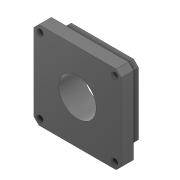
# Autodesk Inventor part: Front cover for servo motor 250 W
Saved by Autodesk Inventor 2020.3 (Build 243373010, 373A)
## iProperties
Created: 2021-04-26
Part Number: Front cover for servo motor 250 W
Material: PBT Plastic
Document SubType Name: Modeling
Designer: marti
Density: 1.31 g/cm^3
Appearance: Smooth - Black
Author: marti
Autodesk Inventor part; units mm, degrees
ref_plane "YZ Plane" through (0, 0, 0) normal (1, 0, 0) x (0, 1, 0)
ref_plane "XZ Plane" through (0, 0, 0) normal (0, 1, 0) x (-1, 0, 0)
ref_plane "XY Plane" through (0, 0, 0) normal (0, 0, 1) x (1, 0, 0)
sketch "Sketch5" plane through (0, 0, 0) normal (0, 0, 1) x (1, 0, 0)
  circle A0 centre (15, -15) radius 1.2295
  circle A1 centre (-15, 15) radius 1.2295
  circle A2 centre (15, 15) radius 1.2295
  circle A3 centre (-15, -15) radius 1.2295
  line L0 (-15.5, -17.5) -> (-17.5, -15.5)
  line L1 (-15.5, -17.5) -> (15.5, -17.5)
  line L2 (17.5, -15.5) -> (15.5, -17.5)
  line L3 (17.5, -15.5) -> (17.5, 15.5)
  line L4 (15.5, 17.5) -> (17.5, 15.5)
  line L5 (15.5, 17.5) -> (-15.5, 17.5)
  line L6 (-17.5, 15.5) -> (-15.5, 17.5)
  line L7 (-17.5, 15.5) -> (-17.5, -15.5)
  circle A4 centre (0, 0) radius 7.5
  dimension "d59" = 15
  constraints: 16 end point, 5 centre point, 1 coincident
  measures "d59" diameter of A4
extrude "Extrusion4" add sketch "Sketch5" against normal mid plane 5
sketch "Sketch6" plane through (0, 0, -2.5) normal (0, 0, -1) x (-1, 0, 0)
  line L0 (14.5, 12.5) -> (14.5, -12.5)
  line L1 (12.5, 14.5) -> (14.5, 12.5)
  line L2 (-12.5, 14.5) -> (12.5, 14.5)
  line L3 (-14.5, 12.5) -> (-12.5, 14.5)
  line L4 (-14.5, -12.5) -> (-14.5, 12.5)
  line L5 (-12.5, -14.5) -> (-14.5, -12.5)
  line L6 (12.5, -14.5) -> (-12.5, -14.5)
  line L7 (14.5, -12.5) -> (12.5, -14.5)
  circle A0 centre (0, 0) radius 7.5 projected
  constraints: 16 end point
extrude "Extrusion5" add sketch "Sketch6" along normal blind 5
body "Solid2"
